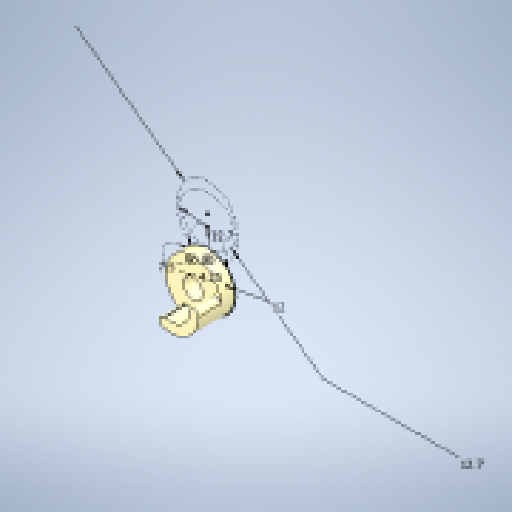
# Autodesk Inventor part: Cam - Shell
Saved by Autodesk Inventor 2023.2 (Build 272271000, 271)
## iProperties
Created: 2024-01-19
Part Number: Cam - Shell
Material: Nylon 6/6
Document SubType Name: Modeling
Designer: Nathan Cai
Density: 1.13 g/cm^3
Appearance: Nylon 6
Mass: 0.456309 g
Surface Area: 4.64642 cm^2
Volume: 0.403814 cm^3
Author: Nathan Cai
Autodesk Inventor part; units mm, degrees
ref_plane "YZ Plane" through (0, 0, 0) normal (1, 0, 0) x (0, 1, 0)
ref_plane "XZ Plane" through (0, 0, 0) normal (0, 1, 0) x (-1, 0, 0)
ref_plane "XY Plane" through (0, 0, 0) normal (0, 0, 1) x (1, 0, 0)
sketch "Sketch1" plane through (0, 0, 0) normal (0, 0, 1) x (1, 0, 0)
  circle A0 centre (0, 0) radius 2.125
  circle A1 centre (0, 0) radius 6
  line L0 (0, 0) -> (0, 6) construction
  line L1 (3.75, 0) -> (3.75, 6)
  line L2 (-3.75, 6) -> (-3.75, 0)
  arc A2 (-3.75, 0) -> (3.75, 0) centre (0, 0) ccw
  arc A3 (3.75, 6) -> (-3.75, 6) centre (0, 6) ccw construction
  line L3 (0, 0) -> (-6, 0) construction
  line L4 (0, 3.75) -> (-6, 3.75)
  line L5 (-6, -3.75) -> (0, -3.75)
  arc A4 (0, -3.75) -> (0, 3.75) centre (0, 0) ccw
  arc A5 (-6, 3.75) -> (-6, -3.75) centre (-6, 0) ccw construction
  circle A6 centre (0, 12.35) radius 6.35 construction
  circle A7 centre (0, 10.1) radius 6.35 construction
  arc A8 (3.75, 4.6837) -> (-4.6837, -3.75) centre (2.5103, -2.5103) ccw
  point P0 (0, 3)
  point P1 (-3, 0)
  point P2 (0, -3.75)
  dimension "d0" = 4.25
  dimension "d3" = 12
  dimension "d4" = 7.5
  dimension "d5" = 7.5
  dimension "d6" = 90
  dimension "d7" = 12.7
  dimension "d8" = 12.7
  constraints: 16 end point, 14 point on circle, 11 tangent, 9 centre point, 4 point on line, 2 coincident, 2 midpoint, 2 parallel, 1 vertical
  measures "d0" diameter of A0
  measures "d3" diameter of A1
  measures "d4" diameter of A3
  measures "d5" diameter of A5
  measures "d6" angle of L0 L3
  measures "d7" diameter of A6
  measures "d8" diameter of A7
extrude "Extrusion1" add sketch "Sketch1" along normal blind 3.175
extrude "Extrusion2" add sketch "Sketch1" along normal blind 7.9375 contours A1 L5 A2 L1
fillet "Fillet1" radius 1 2 edges at (3.75, 4.6837, 5.5563) (-4.6837, -3.75, 5.5563)
equation "\"d4\" = d5"
body "Solid1"
